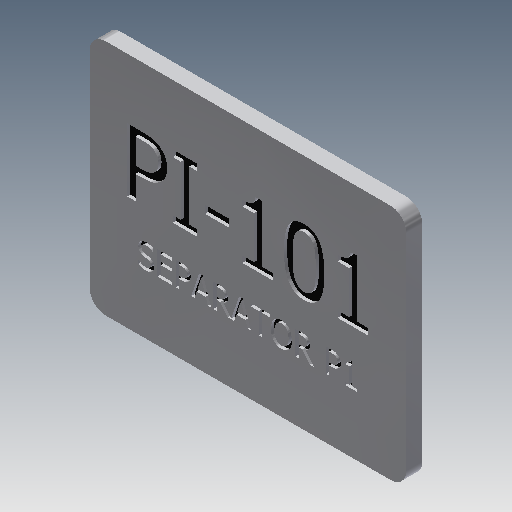
# Autodesk Inventor part: PI-101_Instrument Name Plate
Saved by Autodesk Inventor 2020 (Build 240152000, 152)
## iProperties
Created: 2009-08-11
Part Number: PI-101_Instrument Name Plate
Material: Polyaryletherketone Resin
Document SubType Name: Modeling
Designer: Demir Ali
Mass: 48.5029 g
Surface Area: 174.481 cm^2
Volume: 36.7446 cm^3
Density: 1.32 g/cm^3
Description: Name Plate
Stock Number: NA
Appearance: Smooth - White
Title: Purchased Part
Author: Demir Ali
Revision Number: A
Autodesk Inventor part; units mm, degrees
ref_plane "YZ Plane" through (0, 0, 0) normal (1, 0, 0) x (0, 1, 0)
ref_plane "XZ Plane" through (0, 0, 0) normal (0, 1, 0) x (-1, 0, 0)
ref_plane "XY Plane" through (0, 0, 0) normal (0, 0, 1) x (1, 0, 0)
sketch "Sketch1" plane through (0, 0, 0) normal (0, 0, 1) x (1, 0, 0)
  line L0 (-50, -37.5) -> (50, -37.5)
  line L1 (50, -37.5) -> (50, 37.5)
  line L2 (50, 37.5) -> (-50, 37.5)
  line L3 (-50, 37.5) -> (-50, -37.5)
  point P0 (0, 0)
  point P1 (50, 0)
  point P2 (0, 37.5)
  dimension "d0" = 100
  dimension "d1" = 75
  constraints: 8 end point, 2 midpoint, 2 parallel, 1 horizontal, 1 horizontal alignment, 1 perpendicular, 1 vertical alignment
  measures "d0" distance of L1.end L2.end
  measures "d1" distance of L0.end L1.end
extrude "Extrusion1" add sketch "Sketch1" along normal blind 5
sketch "Sketch2" plane through (0, 0, 5) normal (0, 0, 1) x (1, 0, 0)
  line L0 (-39.7109, 33.8079) -> (39.7109, 33.8079) construction
  line L1 (39.7109, 33.8079) -> (39.7109, -33.8079) construction
  line L2 (39.7109, -33.8079) -> (-39.7109, -33.8079) construction
  line L3 (-39.7109, -33.8079) -> (-39.7109, 33.8079) construction
  line L4 (-50, -37.5) -> (-50, 37.5) projected
  line L5 (50, -37.5) -> (-50, -37.5) projected
  line L6 (50, 37.5) -> (50, -37.5) projected
  line L7 (-50, 37.5) -> (50, 37.5) projected
  spline S0 degree 2 poles (-25.5511, 12.4334) (-25.5511, 11.1368) (-26.4749, 8.8029) (-27.3015, 7.9925) knots 0 0 0 1 2 2 2
  spline S1 degree 2 poles (-27.3015, 7.9925) (-28.3387, 6.9715) (-31.1426, 5.918) (-33.282, 5.918) knots 0 0 0 1 2 2 2
  line L8 (-33.282, 5.918) -> (-35.5348, 5.918)
  line L9 (-35.5348, 5.918) -> (-35.5348, -1.5375)
  line L10 (-35.5348, -1.5375) -> (-38.1929, -1.5375)
  line L11 (-38.1929, -1.5375) -> (-38.1929, 18.4625)
  line L12 (-38.1929, 18.4625) -> (-33.1686, 18.4625)
  spline S2 degree 2 poles (-33.1686, 18.4625) (-31.3857, 18.4625) (-28.8898, 17.8791) (-27.9336, 17.2146) knots 0 0 0 1 2 2 2
  spline S3 degree 2 poles (-27.9336, 17.2146) (-26.8152, 16.4528) (-25.5511, 14.1027) (-25.5511, 12.4334) knots 0 0 0 1 2 2 2
  spline S4 degree 2 poles (-28.3225, 12.3523) (-28.3225, 13.3896) (-29.0357, 14.9131) (-29.765, 15.3993) knots 0 0 0 1 2 2 2
  spline S5 degree 2 poles (-29.765, 15.3993) (-30.3971, 15.8207) (-32.0827, 16.1611) (-33.3306, 16.1611) knots 0 0 0 1 2 2 2
  line L13 (-33.3306, 16.1611) -> (-35.5348, 16.1611)
  line L14 (-35.5348, 16.1611) -> (-35.5348, 8.187)
  line L15 (-35.5348, 8.187) -> (-33.7196, 8.187)
  spline S6 degree 2 poles (-33.7196, 8.187) (-32.0989, 8.187) (-30.1053, 8.7056) (-29.4571, 9.3864) knots 0 0 0 1 2 2 2
  spline S7 degree 2 poles (-29.4571, 9.3864) (-28.8574, 9.986) (-28.3225, 11.3961) (-28.3225, 12.3523) knots 0 0 0 1 2 2 2
  line L16 (-16.0535, -1.5375) -> (-23.8006, -1.5375)
  line L17 (-23.8006, -1.5375) -> (-23.8006, 0.5047)
  line L18 (-23.8006, 0.5047) -> (-21.2561, 0.5047)
  line L19 (-21.2561, 0.5047) -> (-21.2561, 16.4204)
  line L20 (-21.2561, 16.4204) -> (-23.8006, 16.4204)
  line L21 (-23.8006, 16.4204) -> (-23.8006, 18.4625)
  line L22 (-23.8006, 18.4625) -> (-16.0535, 18.4625)
  line L23 (-16.0535, 18.4625) -> (-16.0535, 16.4204)
  line L24 (-16.0535, 16.4204) -> (-18.5981, 16.4204)
  line L25 (-18.5981, 16.4204) -> (-18.5981, 0.5047)
  line L26 (-18.5981, 0.5047) -> (-16.0535, 0.5047)
  line L27 (-16.0535, 0.5047) -> (-16.0535, -1.5375)
  line L28 (-6.0049, 5.999) -> (-13.5737, 5.999)
  line L29 (-13.5737, 5.999) -> (-13.5737, 8.4301)
  line L30 (-13.5737, 8.4301) -> (-6.0049, 8.4301)
  line L31 (-6.0049, 8.4301) -> (-6.0049, 5.999)
  line L32 (7.9822, -1.5375) -> (-1.7747, -1.5375)
  line L33 (-1.7747, -1.5375) -> (-1.7747, 0.5047)
  line L34 (-1.7747, 0.5047) -> (1.8558, 0.5047)
  line L35 (1.8558, 0.5047) -> (1.8558, 13.9082)
  line L36 (1.8558, 13.9082) -> (-1.7747, 13.9082)
  line L37 (-1.7747, 13.9082) -> (-1.7747, 15.7397)
  spline S8 degree 2 poles (-1.7747, 15.7397) (0.2836, 15.7397) (2.2285, 16.9066) (2.3582, 18.5274) knots 0 0 0 1 2 2 2
  line L38 (2.3582, 18.5274) -> (4.4327, 18.5274)
  line L39 (4.4327, 18.5274) -> (4.4327, 0.5047)
  line L40 (4.4327, 0.5047) -> (7.9822, 0.5047)
  line L41 (7.9822, 0.5047) -> (7.9822, -1.5375)
  spline S9 degree 2 poles (24.1086, 8.4625) (24.1086, 3.0817) (20.9806, -1.9589) (17.7229, -1.9589) knots 0 0 0 1 2 2 2
  spline S10 degree 2 poles (17.7229, -1.9589) (14.4165, -1.9589) (11.3209, 3.1789) (11.3209, 8.4463) knots 0 0 0 1 2 2 2
  spline S11 degree 2 poles (11.3209, 8.4463) (11.3209, 13.8596) (14.4489, 18.8677) (17.7229, 18.8677) knots 0 0 0 1 2 2 2
  spline S12 degree 2 poles (17.7229, 18.8677) (21.013, 18.8677) (24.1086, 13.6813) (24.1086, 8.4625) knots 0 0 0 1 2 2 2
  spline S13 degree 2 poles (20.6726, 2.3685) (21.0616, 3.3572) (21.3857, 6.4042) (21.3857, 8.4625) knots 0 0 0 1 2 2 2
  spline S14 degree 2 poles (21.3857, 8.4625) (21.3857, 10.5209) (21.0616, 13.5517) (20.6564, 14.5727) knots 0 0 0 1 2 2 2
  spline S15 degree 2 poles (20.6564, 14.5727) (20.2512, 15.5938) (18.8412, 16.6473) (17.7229, 16.6473) knots 0 0 0 1 2 2 2
  spline S16 degree 2 poles (17.7229, 16.6473) (16.6045, 16.6473) (15.1621, 15.5938) (14.7407, 14.5403) knots 0 0 0 1 2 2 2
  spline S17 degree 2 poles (14.7407, 14.5403) (14.3355, 13.5193) (14.0438, 10.4074) (14.0438, 8.4463) knots 0 0 0 1 2 2 2
  spline S18 degree 2 poles (14.0438, 8.4463) (14.0438, 6.3394) (14.3031, 3.5193) (14.7245, 2.4172) knots 0 0 0 1 2 2 2
  spline S19 degree 2 poles (14.7245, 2.4172) (15.1135, 1.3799) (16.5559, 0.2616) (17.7229, 0.2616) knots 0 0 0 1 2 2 2
  spline S20 degree 2 poles (17.7229, 0.2616) (18.825, 0.2616) (20.2674, 1.315) (20.6726, 2.3685) knots 0 0 0 1 2 2 2
  line L42 (37.9984, -1.5375) -> (28.2415, -1.5375)
  line L43 (28.2415, -1.5375) -> (28.2415, 0.5047)
  line L44 (28.2415, 0.5047) -> (31.872, 0.5047)
  line L45 (31.872, 0.5047) -> (31.872, 13.9082)
  line L46 (31.872, 13.9082) -> (28.2415, 13.9082)
  line L47 (28.2415, 13.9082) -> (28.2415, 15.7397)
  spline S21 degree 2 poles (28.2415, 15.7397) (30.2998, 15.7397) (32.2447, 16.9066) (32.3744, 18.5274) knots 0 0 0 1 2 2 2
  line L48 (32.3744, 18.5274) -> (34.4489, 18.5274)
  line L49 (34.4489, 18.5274) -> (34.4489, 0.5047)
  line L50 (34.4489, 0.5047) -> (37.9984, 0.5047)
  line L51 (37.9984, 0.5047) -> (37.9984, -1.5375)
  spline S22 degree 2 poles (-32.2761, -18.8434) (-33.0906, -18.8434) (-34.2332, -18.5031) (-34.7376, -18.2599) knots 0 0 0 1 2 2 2
  line L52 (-34.7376, -18.2599) -> (-34.7376, -17.0079)
  line L53 (-34.7376, -17.0079) -> (-34.6647, -17.0079)
  spline S23 degree 2 poles (-34.6647, -17.0079) (-34.1724, -17.4698) (-32.9265, -17.9804) (-32.3491, -17.9804) knots 0 0 0 1 2 2 2
  spline S24 degree 2 poles (-32.3491, -17.9804) (-31.5225, -17.9804) (-30.6777, -17.2936) (-30.6777, -16.7283) knots 0 0 0 1 2 2 2
  spline S25 degree 2 poles (-30.6777, -16.7283) (-30.6777, -16.2786) (-31.1214, -15.7194) (-31.6015, -15.5796) knots 0 0 0 1 2 2 2
  spline S26 degree 2 poles (-31.6015, -15.5796) (-31.9479, -15.4824) (-32.5253, -15.3487) (-32.9568, -15.2393) knots 0 0 0 1 2 2 2
  spline S27 degree 2 poles (-32.9568, -15.2393) (-33.3458, -15.136) (-33.9597, -14.826) (-34.1967, -14.5768) knots 0 0 0 1 2 2 2
  spline S28 degree 2 poles (-34.1967, -14.5768) (-34.4277, -14.3276) (-34.6829, -13.6591) (-34.6829, -13.2214) knots 0 0 0 1 2 2 2
  spline S29 degree 2 poles (-34.6829, -13.2214) (-34.6829, -12.3098) (-33.2607, -11.076) (-32.1607, -11.076) knots 0 0 0 1 2 2 2
  spline S30 degree 2 poles (-32.1607, -11.076) (-31.5286, -11.076) (-30.4103, -11.3252) (-29.9301, -11.5622) knots 0 0 0 1 2 2 2
  line L54 (-29.9301, -11.5622) -> (-29.9301, -12.7535)
  line L55 (-29.9301, -12.7535) -> (-30.003, -12.7535)
  spline S31 degree 2 poles (-30.003, -12.7535) (-30.3616, -12.4253) (-31.4799, -11.939) (-32.0938, -11.939) knots 0 0 0 1 2 2 2
  spline S32 degree 2 poles (-32.0938, -11.939) (-32.7867, -11.939) (-33.6436, -12.5894) (-33.6436, -13.1181) knots 0 0 0 1 2 2 2
  spline S33 degree 2 poles (-33.6436, -13.1181) (-33.6436, -13.5922) (-33.1392, -14.1574) (-32.6651, -14.2851) knots 0 0 0 1 2 2 2
  spline S34 degree 2 poles (-32.6651, -14.2851) (-32.3491, -14.3702) (-31.4313, -14.589) (-31.1274, -14.6801) knots 0 0 0 1 2 2 2
  spline S35 degree 2 poles (-31.1274, -14.6801) (-30.3556, -14.9172) (-29.6384, -15.8714) (-29.6384, -16.5703) knots 0 0 0 1 2 2 2
  spline S36 degree 2 poles (-29.6384, -16.5703) (-29.6384, -17.014) (-29.997, -17.8649) (-30.3191, -18.1627) knots 0 0 0 1 2 2 2
  spline S37 degree 2 poles (-30.3191, -18.1627) (-30.6777, -18.4909) (-31.5893, -18.8434) (-32.2761, -18.8434) knots 0 0 0 1 2 2 2
  line L56 (-28.6234, -18.7097) -> (-28.6234, -11.2097)
  line L57 (-28.6234, -11.2097) -> (-23.9313, -11.2097)
  line L58 (-23.9313, -11.2097) -> (-23.9313, -12.0971)
  line L59 (-23.9313, -12.0971) -> (-27.6266, -12.0971)
  line L60 (-27.6266, -12.0971) -> (-27.6266, -14.1514)
  line L61 (-27.6266, -14.1514) -> (-24.1805, -14.1514)
  line L62 (-24.1805, -14.1514) -> (-24.1805, -15.0387)
  line L63 (-24.1805, -15.0387) -> (-27.6266, -15.0387)
  line L64 (-27.6266, -15.0387) -> (-27.6266, -17.8223)
  line L65 (-27.6266, -17.8223) -> (-23.9313, -17.8223)
  line L66 (-23.9313, -17.8223) -> (-23.9313, -18.7097)
  line L67 (-23.9313, -18.7097) -> (-28.6234, -18.7097)
  spline S38 degree 2 poles (-18.0966, -13.4706) (-18.0966, -13.9569) (-18.4431, -14.8321) (-18.753, -15.136) knots 0 0 0 1 2 2 2
  spline S39 degree 2 poles (-18.753, -15.136) (-19.142, -15.5189) (-20.1935, -15.9139) (-20.9957, -15.9139) knots 0 0 0 1 2 2 2
  line L68 (-20.9957, -15.9139) -> (-21.8406, -15.9139)
  line L69 (-21.8406, -15.9139) -> (-21.8406, -18.7097)
  line L70 (-21.8406, -18.7097) -> (-22.8373, -18.7097)
  line L71 (-22.8373, -18.7097) -> (-22.8373, -11.2097)
  line L72 (-22.8373, -11.2097) -> (-20.9532, -11.2097)
  spline S40 degree 2 poles (-20.9532, -11.2097) (-20.2846, -11.2097) (-19.3487, -11.4285) (-18.9901, -11.6777) knots 0 0 0 1 2 2 2
  spline S41 degree 2 poles (-18.9901, -11.6777) (-18.5707, -11.9633) (-18.0966, -12.8446) (-18.0966, -13.4706) knots 0 0 0 1 2 2 2
  spline S42 degree 2 poles (-19.1359, -13.501) (-19.1359, -13.112) (-19.4034, -12.5407) (-19.6769, -12.3584) knots 0 0 0 1 2 2 2
  spline S43 degree 2 poles (-19.6769, -12.3584) (-19.9139, -12.2004) (-20.546, -12.0727) (-21.014, -12.0727) knots 0 0 0 1 2 2 2
  line L73 (-21.014, -12.0727) -> (-21.8406, -12.0727)
  line L74 (-21.8406, -12.0727) -> (-21.8406, -15.063)
  line L75 (-21.8406, -15.063) -> (-21.1598, -15.063)
  spline S44 degree 2 poles (-21.1598, -15.063) (-20.5521, -15.063) (-19.8045, -14.8685) (-19.5614, -14.6133) knots 0 0 0 1 2 2 2
  spline S45 degree 2 poles (-19.5614, -14.6133) (-19.3365, -14.3884) (-19.1359, -13.8596) (-19.1359, -13.501) knots 0 0 0 1 2 2 2
  line L76 (-17.9568, -18.7097) -> (-15.4285, -11.2097)
  line L77 (-15.4285, -11.2097) -> (-14.2008, -11.2097)
  line L78 (-14.2008, -11.2097) -> (-11.6724, -18.7097)
  line L79 (-11.6724, -18.7097) -> (-12.7239, -18.7097)
  line L80 (-12.7239, -18.7097) -> (-13.4046, -16.6129)
  line L81 (-13.4046, -16.6129) -> (-16.2672, -16.6129)
  line L82 (-16.2672, -16.6129) -> (-16.9479, -18.7097)
  line L83 (-16.9479, -18.7097) -> (-17.9568, -18.7097)
  line L84 (-13.6781, -15.762) -> (-14.8389, -12.2308)
  line L85 (-14.8389, -12.2308) -> (-15.9937, -15.762)
  line L86 (-15.9937, -15.762) -> (-13.6781, -15.762)
  line L87 (-5.157, -18.7097) -> (-6.4516, -18.7097)
  line L88 (-6.4516, -18.7097) -> (-8.8219, -15.7255)
  line L89 (-8.8219, -15.7255) -> (-9.9645, -15.7255)
  line L90 (-9.9645, -15.7255) -> (-9.9645, -18.7097)
  line L91 (-9.9645, -18.7097) -> (-10.9613, -18.7097)
  line L92 (-10.9613, -18.7097) -> (-10.9613, -11.2097)
  line L93 (-10.9613, -11.2097) -> (-9.0286, -11.2097)
  spline S46 degree 2 poles (-9.0286, -11.2097) (-8.3843, -11.2097) (-7.5152, -11.3495) (-7.1201, -11.6048) knots 0 0 0 1 2 2 2
  spline S47 degree 2 poles (-7.1201, -11.6048) (-6.7251, -11.86) (-6.2692, -12.6562) (-6.2692, -13.2458) knots 0 0 0 1 2 2 2
  spline S48 degree 2 poles (-6.2692, -13.2458) (-6.2692, -14.0663) (-7.108, -15.1785) (-7.8252, -15.4459) knots 0 0 0 1 2 2 2
  line L94 (-7.8252, -15.4459) -> (-5.157, -18.7097)
  spline S49 degree 2 poles (-7.3086, -13.3248) (-7.3086, -12.9966) (-7.5395, -12.4921) (-7.7826, -12.328) knots 0 0 0 1 2 2 2
  spline S50 degree 2 poles (-7.7826, -12.328) (-7.9953, -12.1882) (-8.5606, -12.0727) (-8.9739, -12.0727) knots 0 0 0 1 2 2 2
  line L95 (-8.9739, -12.0727) -> (-9.9645, -12.0727)
  line L96 (-9.9645, -12.0727) -> (-9.9645, -14.8928)
  line L97 (-9.9645, -14.8928) -> (-9.0893, -14.8928)
  spline S51 degree 2 poles (-9.0893, -14.8928) (-8.6578, -14.8928) (-7.971, -14.7409) (-7.734, -14.5039) knots 0 0 0 1 2 2 2
  spline S52 degree 2 poles (-7.734, -14.5039) (-7.5152, -14.2972) (-7.3086, -13.7138) (-7.3086, -13.3248) knots 0 0 0 1 2 2 2
  line L98 (-5.3697, -18.7097) -> (-2.8414, -11.2097)
  line L99 (-2.8414, -11.2097) -> (-1.6137, -11.2097)
  line L100 (-1.6137, -11.2097) -> (0.9147, -18.7097)
  line L101 (0.9147, -18.7097) -> (-0.1368, -18.7097)
  line L102 (-0.1368, -18.7097) -> (-0.8175, -16.6129)
  line L103 (-0.8175, -16.6129) -> (-3.6801, -16.6129)
  line L104 (-3.6801, -16.6129) -> (-4.3608, -18.7097)
  line L105 (-4.3608, -18.7097) -> (-5.3697, -18.7097)
  line L106 (-1.091, -15.762) -> (-2.2518, -12.2308)
  line L107 (-2.2518, -12.2308) -> (-3.4066, -15.762)
  line L108 (-3.4066, -15.762) -> (-1.091, -15.762)
  line L109 (3.3762, -18.7097) -> (3.3762, -12.0971)
  line L110 (3.3762, -12.0971) -> (0.86, -12.0971)
  line L111 (0.86, -12.0971) -> (0.86, -11.2097)
  line L112 (0.86, -11.2097) -> (6.8892, -11.2097)
  line L113 (6.8892, -11.2097) -> (6.8892, -12.0971)
  line L114 (6.8892, -12.0971) -> (4.373, -12.0971)
  line L115 (4.373, -12.0971) -> (4.373, -18.7097)
  line L116 (4.373, -18.7097) -> (3.3762, -18.7097)
  spline S53 degree 2 poles (12.9548, -12.0667) (13.3803, -12.565) (13.8543, -14.0237) (13.8543, -14.9597) knots 0 0 0 1 2 2 2
  spline S54 degree 2 poles (13.8543, -14.9597) (13.8543, -15.8714) (13.3924, -17.3483) (12.9548, -17.8467) knots 0 0 0 1 2 2 2
  spline S55 degree 2 poles (12.9548, -17.8467) (12.4929, -18.3693) (11.2713, -18.8677) (10.5359, -18.8677) knots 0 0 0 1 2 2 2
  spline S56 degree 2 poles (10.5359, -18.8677) (9.7761, -18.8677) (8.5606, -18.3511) (8.1169, -17.8467) knots 0 0 0 1 2 2 2
  spline S57 degree 2 poles (8.1169, -17.8467) (7.6854, -17.3483) (7.2235, -15.8835) (7.2235, -14.9597) knots 0 0 0 1 2 2 2
  spline S58 degree 2 poles (7.2235, -14.9597) (7.2235, -14.0176) (7.6914, -12.5833) (8.123, -12.0667) knots 0 0 0 1 2 2 2
  spline S59 degree 2 poles (8.123, -12.0667) (8.5606, -11.5683) (9.7822, -11.0517) (10.5359, -11.0517) knots 0 0 0 1 2 2 2
  spline S60 degree 2 poles (10.5359, -11.0517) (11.3017, -11.0517) (12.5294, -11.5865) (12.9548, -12.0667) knots 0 0 0 1 2 2 2
  spline S61 degree 2 poles (12.815, -14.9597) (12.815, -14.2182) (12.4929, -13.0695) (12.2012, -12.6927) knots 0 0 0 1 2 2 2
  spline S62 degree 2 poles (12.2012, -12.6927) (11.9034, -12.3037) (11.0646, -11.9147) (10.5419, -11.9147) knots 0 0 0 1 2 2 2
  spline S63 degree 2 poles (10.5419, -11.9147) (10.001, -11.9147) (9.1866, -12.2915) (8.8766, -12.6927) knots 0 0 0 1 2 2 2
  spline S64 degree 2 poles (8.8766, -12.6927) (8.5788, -13.0756) (8.2628, -14.2304) (8.2628, -14.9597) knots 0 0 0 1 2 2 2
  spline S65 degree 2 poles (8.2628, -14.9597) (8.2628, -16.4366) (9.5026, -18.0047) (10.5419, -18.0047) knots 0 0 0 1 2 2 2
  spline S66 degree 2 poles (10.5419, -18.0047) (11.5812, -18.0047) (12.815, -16.4366) (12.815, -14.9597) knots 0 0 0 1 2 2 2
  line L117 (20.7526, -18.7097) -> (19.4581, -18.7097)
  line L118 (19.4581, -18.7097) -> (17.0877, -15.7255)
  line L119 (17.0877, -15.7255) -> (15.9451, -15.7255)
  line L120 (15.9451, -15.7255) -> (15.9451, -18.7097)
  line L121 (15.9451, -18.7097) -> (14.9483, -18.7097)
  line L122 (14.9483, -18.7097) -> (14.9483, -11.2097)
  line L123 (14.9483, -11.2097) -> (16.8811, -11.2097)
  spline S67 degree 2 poles (16.8811, -11.2097) (17.5253, -11.2097) (18.3944, -11.3495) (18.7895, -11.6048) knots 0 0 0 1 2 2 2
  spline S68 degree 2 poles (18.7895, -11.6048) (19.1846, -11.86) (19.6404, -12.6562) (19.6404, -13.2458) knots 0 0 0 1 2 2 2
  spline S69 degree 2 poles (19.6404, -13.2458) (19.6404, -14.0663) (18.8017, -15.1785) (18.0845, -15.4459) knots 0 0 0 1 2 2 2
  line L124 (18.0845, -15.4459) -> (20.7526, -18.7097)
  spline S70 degree 2 poles (18.6011, -13.3248) (18.6011, -12.9966) (18.3701, -12.4921) (18.127, -12.328) knots 0 0 0 1 2 2 2
  spline S71 degree 2 poles (18.127, -12.328) (17.9143, -12.1882) (17.3491, -12.0727) (16.9358, -12.0727) knots 0 0 0 1 2 2 2
  line L125 (16.9358, -12.0727) -> (15.9451, -12.0727)
  line L126 (15.9451, -12.0727) -> (15.9451, -14.8928)
  line L127 (15.9451, -14.8928) -> (16.8203, -14.8928)
  spline S72 degree 2 poles (16.8203, -14.8928) (17.2518, -14.8928) (17.9386, -14.7409) (18.1756, -14.5039) knots 0 0 0 1 2 2 2
  spline S73 degree 2 poles (18.1756, -14.5039) (18.3944, -14.2972) (18.6011, -13.7138) (18.6011, -13.3248) knots 0 0 0 1 2 2 2
  spline S74 degree 2 poles (29.3102, -13.4706) (29.3102, -13.9569) (28.9637, -14.8321) (28.6538, -15.136) knots 0 0 0 1 2 2 2
  spline S75 degree 2 poles (28.6538, -15.136) (28.2648, -15.5189) (27.2133, -15.9139) (26.4111, -15.9139) knots 0 0 0 1 2 2 2
  line L128 (26.4111, -15.9139) -> (25.5662, -15.9139)
  line L129 (25.5662, -15.9139) -> (25.5662, -18.7097)
  line L130 (25.5662, -18.7097) -> (24.5695, -18.7097)
  line L131 (24.5695, -18.7097) -> (24.5695, -11.2097)
  line L132 (24.5695, -11.2097) -> (26.4536, -11.2097)
  spline S76 degree 2 poles (26.4536, -11.2097) (27.1222, -11.2097) (28.0581, -11.4285) (28.4167, -11.6777) knots 0 0 0 1 2 2 2
  spline S77 degree 2 poles (28.4167, -11.6777) (28.8361, -11.9633) (29.3102, -12.8446) (29.3102, -13.4706) knots 0 0 0 1 2 2 2
  spline S78 degree 2 poles (28.2709, -13.501) (28.2709, -13.112) (28.0034, -12.5407) (27.7299, -12.3584) knots 0 0 0 1 2 2 2
  spline S79 degree 2 poles (27.7299, -12.3584) (27.4929, -12.2004) (26.8608, -12.0727) (26.3928, -12.0727) knots 0 0 0 1 2 2 2
  line L133 (26.3928, -12.0727) -> (25.5662, -12.0727)
  line L134 (25.5662, -12.0727) -> (25.5662, -15.063)
  line L135 (25.5662, -15.063) -> (26.247, -15.063)
  spline S80 degree 2 poles (26.247, -15.063) (26.8547, -15.063) (27.6023, -14.8685) (27.8454, -14.6133) knots 0 0 0 1 2 2 2
  spline S81 degree 2 poles (27.8454, -14.6133) (28.0703, -14.3884) (28.2709, -13.8596) (28.2709, -13.501) knots 0 0 0 1 2 2 2
  line L136 (34.294, -18.7097) -> (30.6351, -18.7097)
  line L137 (30.6351, -18.7097) -> (30.6351, -17.9439)
  line L138 (30.6351, -17.9439) -> (31.9966, -17.9439)
  line L139 (31.9966, -17.9439) -> (31.9966, -12.9176)
  line L140 (31.9966, -12.9176) -> (30.6351, -12.9176)
  line L141 (30.6351, -12.9176) -> (30.6351, -12.2308)
  spline S82 degree 2 poles (30.6351, -12.2308) (31.407, -12.2308) (32.1363, -11.7932) (32.185, -11.1854) knots 0 0 0 1 2 2 2
  line L142 (32.185, -11.1854) -> (32.9629, -11.1854)
  line L143 (32.9629, -11.1854) -> (32.9629, -17.9439)
  line L144 (32.9629, -17.9439) -> (34.294, -17.9439)
  line L145 (34.294, -17.9439) -> (34.294, -18.7097)
  point P0 (0, 0)
  point P1 (0, 33.8079)
  point P2 (-39.7109, 0)
  constraints: 2 midpoint, 1 horizontal alignment, 1 vertical alignment, 2 other
emboss "Emboss1" sketch "Sketch2" operation cut depth 1 direction (0, 0, -1) contours S0 S1 L8 L9 L10 L11 L12 S2 S3 | L16 L17 L18 L19 L20 L21 L22 L23 L24 L25 L26 L27 | L28 L29 L30 L31 | L32 L33 L34 L35 L36 L37 S8 L38 L39 L40 L41 | S9 S10 S11 S12 | L42 L43 L44 L45 L46 L47 S21 L48 L49 L50 L51 | S22 L52 L53 S23 S24 S25 S26 S27 S28 S29 S30 L54 L55 S31 S32 S33 S34 S35 S36 S37 | L56 L57 L58 L59 L60 L61 L62 L63 L64 L65 L66 L67 | S38 S39 L68 L69 L70 L71 L72 S40 S41 | L76 L77 L78 L79 L80 L81 L82 L83 | L87 L98 L94 | L94 L98 L99 L100 L101 L102 L103 L104 L105 | L87 L88 L89 L90 L91 L92 L93 S46 S47 S48 L94 L98 | L109 L110 L111 L112 L113 L114 L115 L116 | S53 S54 S55 S56 S57 S58 S59 S60 | L117 L118 L119 L120 L121 L122 L123 S67 S68 S69 L124 | S74 S75 L128 L129 L130 L131 L132 S76 S77 | L136 L137 L138 L139 L140 L141 S82 L142 L143 L144 L145
fillet "Fillet1" radius 5 4 edges at (-50, 37.5, 2.5) (50, 37.5, 2.5) (-50, -37.5, 2.5) (50, -37.5, 2.5)
body "Solid1"
